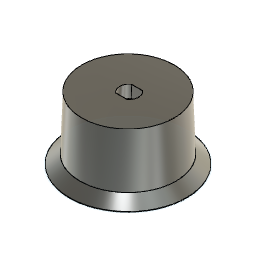
Cup_Tray v4 (Autodesk Fusion 360 design; units mm, degrees)
Autodesk Fusion 360 part; units mm, degrees
sketch "Sketch1" plane through (0, 0, 0) normal (0, 0, 1) x (1, 0, 0)
  circle A0 centre (0, 0) radius 15.5
  dimension "d1" = 31
  constraint coincident A0.centre origin
  measures "d1" diameter of A0
extrude "Extrude1" add sketch "Sketch1" along normal blind 2.5 draft -50
sketch "Sketch2" plane through (0, 0, 2.5) normal (0, 0, 1) x (-1, 0, 0)
  circle A0 centre (0, 0) radius 12.520616
  circle A1 centre (0, 0) radius 12.5
  dimension "d4" = 25
  constraint coincident A0.centre A1.centre
  measures "d4" diameter of A1
extrude "Extrude2" add sketch "Sketch2" along normal blind 14 draft -2 contours A0 A1 picked at (-3.532337, 1.230172)
sketch "Sketch3" plane through (0, 0, 0) normal (0, 0, -1) x (1, 0, 0)
  circle A0 centre (0, 0) radius 15.5
sketch "Sketch4" plane through (0, 0, 0) normal (0, 0, -1) x (1, 0, 0)
  circle A0 centre (0, 0) radius 9.5
  dimension "d7" = 19
  constraint coincident A0.centre origin
  measures "d7" diameter of A0
extrude "Extrude3" cut sketch "Sketch4" against normal blind 13
fillet "Fillet1" radius 7 1 faces at (2.084686, 1.003932, 13)
sketch "Sketch5" plane through (0, 0, 16.5) normal (0, 0, 1) x (-1, 0, 0)
  circle A0 centre (0, 0) radius 12.011109
  arc A1 (-1.650258, 1.92644) -> (-1.650258, -2.07356) centre (-0.258807, -0.07356) ccw
  line L0 (-1.650258, -2.07356) -> (1.241193, -2.07356)
  arc A2 (1.241193, -2.07356) -> (1.241193, 1.92644) centre (-0.258807, -0.07356) ccw
  line L1 (1.241193, 1.92644) -> (-1.650258, 1.92644)
  dimension "d11" = 5
  dimension "d12" = 4
  constraint horizontal L1
  constraint parallel L0 L1
  constraint concentric A1 A2
  constraint equal L0 L1
  measures "d11" diameter of A2
extrude "Extrude4" cut sketch "Sketch5" against normal through all draft 5 contours A1 L0 A2 L1 picked at (-0.355227, -0.014168)
fillet "Fillet2" radius 0.1 1 edges at (-14.451074, -5.605039, 0)
